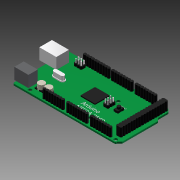
# Autodesk Inventor part: ArduinoMEGA2560
Saved by Autodesk Inventor 2012 (Build 160160000, 160)
## iProperties
Created: 2012-05-11
Part Number: ArduinoMEGA2560
Material: ABS Plastic
Document SubType Name: Modeling
Mass: 17.2903 g
Surface Area: 176.309 cm^2
Volume: 16.3116 cm^3
Density: 1.06 g/cm^3
Autodesk Inventor part; units mm, degrees
(part 1 of 2)
ref_plane "YZ Plane" through (0, 0, 0) normal (1, 0, 0) x (0, 1, 0)
ref_plane "XZ Plane" through (0, 0, 0) normal (0, 1, 0) x (-1, 0, 0)
sketch "Sketch1" plane through (0, 0, 0) normal (0, 0, 1) x (1, 0, 0)
  line L0 (96.5199, 53.3399) -> (99.0599, 50.7999)
  line L1 (99.0599, 40.6399) -> (101.5999, 38.0999)
  line L2 (101.5999, 38.0999) -> (101.5999, 3.81)
  line L3 (101.5999, 3.81) -> (99.0599, 1.27)
  line L4 (99.0599, 1.27) -> (99.0599, 1)
  arc A0 (98.0599, 0) -> (99.0599, 1) centre (98.0599, 1) ccw
  line L5 (98.0599, 0) -> (1, 0)
  arc A1 (0, 1) -> (1, 0) centre (1, 1) ccw
  line L6 (0, 1) -> (0, 52.3399)
  arc A2 (1, 53.3399) -> (0, 52.3399) centre (1, 52.3399) ccw
  line L7 (1, 53.3399) -> (96.5199, 53.3399)
  line L8 (99.0599, 50.7999) -> (99.0599, 40.6399)
  circle A3 centre (96.52, 2.54) radius 1.6
  circle A4 centre (15.24, 50.7999) radius 1.6
  circle A5 centre (90.17, 50.7999) radius 1.6
  circle A6 centre (13.97, 2.54) radius 1.6
  circle A7 centre (66.04, 35.5599) radius 1.6
  circle A8 centre (66.04, 7.62) radius 1.6
  point P0 (0, 0)
  dimension "d51" = 3.2
  dimension "d52" = 53.3399
  dimension "d53" = 101.5999
  dimension "d56" = 13.97
  dimension "d57" = 15.24
  dimension "d58" = 66.04
  dimension "d59" = 90.17
  dimension "d60" = 96.5199
  dimension "d61" = 2.54
  dimension "d62" = 50.7999
  dimension "d63" = 7.62
  dimension "d64" = 27.9399
  dimension "d65" = 98.0599
  dimension "d66" = 1
  dimension "d67" = 45
  dimension "d68" = 2.54
  dimension "d69" = 2.54
  dimension "d73" = 1.27
  dimension "d74" = 12.7
  constraints: 18 end point, 9 centre point, 7 equal radius, 7 tangent, 6 point on circle, 2 horizontal alignment, 2 parallel, 2 point on line, 1 horizontal, 1 perpendicular, 1 vertical, 1 vertical alignment
  measures "d51" diameter of A4
  measures "d52" distance between parallel lines of L5 L7
  measures "d53" distance between parallel lines of L2 L6
  measures "d56" distance from line of A6.centre L6
  measures "d57" distance from line of A4.centre L6
  measures "d58" distance from line of A7.centre L6
  measures "d59" distance from line of A5.centre L6
  measures "d60" distance from line of A3.centre L6
  measures "d61" distance from line of A6.centre L5
  measures "d62" distance from line of A4.centre L5
  measures "d63" distance from line of L5 A8.centre
  measures "d64" distance of A7.centre A8.centre
  measures "d65" distance from line of L6 A0.centre
  measures "d66" radius of A0
  measures "d67" angle of L7 L0
  measures "d68" horizontal distance of L0.start L0.end
  measures "d69" horizontal distance of L1.start L1.end
  measures "d73" distance from line of L3.end L5
  measures "d74" distance from line of L7 L1.start
extrude "PCB" add sketch "Sketch1" against normal blind 1.6
sketch "Sketch3" plane through (0, 0, 0) normal (0, 0, 1) x (1, 0, 0)
  arc A0 (21.844, 24.257) -> (21.844, 27.813) centre (21.844, 26.035) ccw
  arc A1 (21.844, 23.749) -> (21.844, 28.321) centre (21.844, 26.035) ccw
  arc A2 (14.986, 28.321) -> (14.986, 23.749) centre (14.986, 26.035) ccw
  arc A3 (14.986, 27.813) -> (14.986, 24.257) centre (14.986, 26.035) ccw
  line L0 (14.986, 24.257) -> (21.844, 24.257)
  line L1 (21.844, 27.813) -> (14.986, 27.813)
  line L2 (14.986, 23.749) -> (21.844, 23.749)
  line L3 (21.844, 28.321) -> (14.986, 28.321)
  line L4 (97.155, 6.35) -> (93.345, 6.35)
  arc A4 (97.155, 8.8519) -> (97.155, 8.9281) centre (97.155, 8.89) ccw
  line L5 (97.155, 8.89) -> (93.345, 8.89)
  line L6 (97.155, 11.43) -> (93.345, 11.43)
  line L7 (97.155, 13.97) -> (93.345, 13.97)
  line L8 (97.155, 16.51) -> (93.345, 16.51)
  line L9 (97.155, 19.05) -> (93.345, 19.05)
  line L10 (97.155, 21.59) -> (93.345, 21.59)
  line L11 (97.155, 24.13) -> (93.345, 24.13)
  line L12 (97.155, 26.67) -> (93.345, 26.67)
  line L13 (97.155, 29.21) -> (93.345, 29.21)
  line L14 (97.155, 31.75) -> (93.345, 31.75)
  line L15 (97.155, 34.29) -> (93.345, 34.29)
  line L16 (97.155, 36.83) -> (93.345, 36.83)
  line L17 (97.155, 39.37) -> (93.345, 39.37)
  line L18 (97.155, 41.91) -> (93.345, 41.91)
  line L19 (97.155, 44.45) -> (93.345, 44.45)
  line L20 (97.155, 46.99) -> (93.345, 46.99)
  line L21 (97.155, 49.53) -> (93.345, 49.53)
  line L22 (93.345, 36.83) -> (92.71, 36.195)
  line L23 (92.71, 34.925) -> (92.71, 36.195)
  line L24 (93.345, 34.29) -> (92.71, 34.925)
  line L25 (93.345, 34.29) -> (92.71, 33.655)
  line L26 (92.71, 32.385) -> (92.71, 33.655)
  line L27 (93.345, 31.75) -> (92.71, 32.385)
  line L28 (93.345, 31.75) -> (92.71, 31.115)
  line L29 (92.71, 29.845) -> (92.71, 31.115)
  line L30 (93.345, 29.21) -> (92.71, 29.845)
  line L31 (93.345, 29.21) -> (92.71, 28.575)
  line L32 (92.71, 27.305) -> (92.71, 28.575)
  line L33 (93.345, 26.67) -> (92.71, 27.305)
  line L34 (93.345, 26.67) -> (92.71, 26.035)
  line L35 (92.71, 24.765) -> (92.71, 26.035)
  line L36 (93.345, 24.13) -> (92.71, 24.765)
  line L37 (93.345, 24.13) -> (92.71, 23.495)
  line L38 (92.71, 22.225) -> (92.71, 23.495)
  line L39 (93.345, 21.59) -> (92.71, 22.225)
  line L40 (93.345, 21.59) -> (92.71, 20.955)
  line L41 (92.71, 19.685) -> (92.71, 20.955)
  line L42 (93.345, 19.05) -> (92.71, 19.685)
  line L43 (93.345, 19.05) -> (92.71, 18.415)
  line L44 (92.71, 17.145) -> (92.71, 18.415)
  line L45 (93.345, 16.51) -> (92.71, 17.145)
  line L46 (92.71, 15.875) -> (93.345, 16.51)
  line L47 (92.71, 15.875) -> (92.71, 14.605)
  line L48 (93.345, 13.97) -> (92.71, 14.605)
  line L49 (92.71, 13.335) -> (93.345, 13.97)
  line L50 (92.71, 13.335) -> (92.71, 12.065)
  line L51 (93.345, 11.43) -> (92.71, 12.065)
  line L52 (93.345, 11.43) -> (92.71, 10.795)
  line L53 (92.71, 9.525) -> (92.71, 10.795)
  line L54 (93.345, 8.89) -> (92.71, 9.525)
  line L55 (93.345, 8.89) -> (92.71, 8.255)
  line L56 (92.71, 6.985) -> (92.71, 8.255)
  line L57 (93.345, 6.35) -> (92.71, 6.985)
  line L58 (97.79, 6.985) -> (97.155, 6.35)
  line L59 (97.79, 6.985) -> (97.79, 8.255)
  arc A5 (97.1819, 8.9169) -> (97.1281, 8.8631) centre (97.155, 8.89) ccw
  line L60 (97.155, 8.89) -> (97.79, 8.255)
  arc A6 (97.1281, 8.8631) -> (97.1819, 8.8631) centre (97.155, 8.89) ccw
  line L61 (97.79, 9.525) -> (97.155, 8.89)
  line L62 (97.79, 9.525) -> (97.79, 10.795)
  line L63 (97.155, 11.43) -> (97.79, 10.795)
  line L64 (97.79, 12.065) -> (97.155, 11.43)
  line L65 (97.79, 12.065) -> (97.79, 13.335)
  line L66 (97.155, 13.97) -> (97.79, 13.335)
  line L67 (97.79, 14.605) -> (97.155, 13.97)
  line L68 (97.79, 14.605) -> (97.79, 15.875)
  line L69 (97.155, 16.51) -> (97.79, 15.875)
  line L70 (97.79, 17.145) -> (97.155, 16.51)
  line L71 (97.79, 17.145) -> (97.79, 18.415)
  line L72 (97.155, 19.05) -> (97.79, 18.415)
  line L73 (97.79, 19.685) -> (97.155, 19.05)
  line L74 (97.79, 19.685) -> (97.79, 20.955)
  line L75 (97.155, 21.59) -> (97.79, 20.955)
  line L76 (97.155, 21.59) -> (97.79, 22.225)
  line L77 (97.79, 23.495) -> (97.79, 22.225)
  line L78 (97.155, 24.13) -> (97.79, 23.495)
  line L79 (97.79, 24.765) -> (97.155, 24.13)
  line L80 (97.79, 26.035) -> (97.79, 24.765)
  line L81 (97.155, 26.67) -> (97.79, 26.035)
  line L82 (97.79, 27.305) -> (97.155, 26.67)
  line L83 (97.79, 28.575) -> (97.79, 27.305)
  line L84 (97.155, 29.21) -> (97.79, 28.575)
  line L85 (97.79, 29.845) -> (97.155, 29.21)
  line L86 (97.79, 31.115) -> (97.79, 29.845)
  line L87 (97.155, 31.75) -> (97.79, 31.115)
  line L88 (97.79, 32.385) -> (97.155, 31.75)
  line L89 (97.79, 33.655) -> (97.79, 32.385)
  line L90 (97.155, 34.29) -> (97.79, 33.655)
  line L91 (97.79, 34.925) -> (97.155, 34.29)
  line L92 (97.79, 36.195) -> (97.79, 34.925)
  line L93 (97.155, 36.83) -> (97.79, 36.195)
  line L94 (97.79, 37.465) -> (97.155, 36.83)
  line L95 (97.79, 38.735) -> (97.79, 37.465)
  line L96 (97.155, 39.37) -> (97.79, 38.735)
  line L97 (97.79, 40.005) -> (97.155, 39.37)
  line L98 (97.79, 41.275) -> (97.79, 40.005)
  line L99 (97.155, 41.91) -> (97.79, 41.275)
  line L100 (97.79, 42.545) -> (97.155, 41.91)
  line L101 (97.79, 43.815) -> (97.79, 42.545)
  line L102 (97.155, 44.45) -> (97.79, 43.815)
  line L103 (97.79, 45.085) -> (97.155, 44.45)
  line L104 (97.79, 46.355) -> (97.79, 45.085)
  line L105 (97.155, 46.99) -> (97.79, 46.355)
  line L106 (97.79, 47.625) -> (97.155, 46.99)
  line L107 (97.79, 48.895) -> (97.79, 47.625)
  line L108 (97.155, 49.53) -> (97.79, 48.895)
  line L109 (97.79, 50.165) -> (97.155, 49.53)
  line L110 (97.79, 51.435) -> (97.79, 50.165)
  line L111 (97.155, 52.07) -> (97.79, 51.435)
  line L112 (93.345, 52.07) -> (97.155, 52.07)
  line L113 (92.71, 37.465) -> (93.345, 36.83)
  line L114 (92.71, 38.735) -> (92.71, 37.465)
  line L115 (93.345, 39.37) -> (92.71, 38.735)
  line L116 (92.71, 40.005) -> (93.345, 39.37)
  line L117 (92.71, 41.275) -> (92.71, 40.005)
  line L118 (93.345, 41.91) -> (92.71, 41.275)
  line L119 (92.71, 42.545) -> (93.345, 41.91)
  line L120 (92.71, 43.815) -> (92.71, 42.545)
  line L121 (93.345, 44.45) -> (92.71, 43.815)
  line L122 (92.71, 45.085) -> (93.345, 44.45)
  line L123 (92.71, 46.355) -> (92.71, 45.085)
  line L124 (93.345, 46.99) -> (92.71, 46.355)
  line L125 (92.71, 47.625) -> (93.345, 46.99)
  line L126 (92.71, 48.895) -> (92.71, 47.625)
  line L127 (93.345, 49.53) -> (92.71, 48.895)
  line L128 (92.71, 50.165) -> (93.345, 49.53)
  line L129 (92.71, 51.435) -> (92.71, 50.165)
  line L130 (93.345, 52.07) -> (92.71, 51.435)
  line L131 (8.763, 27.3304) -> (9.525, 27.3304)
  line L132 (8.763, 24.4348) -> (8.763, 27.3304)
  line L133 (9.525, 24.4348) -> (8.763, 24.4348)
  line L134 (9.525, 27.3304) -> (9.525, 24.4348)
  line L135 (26.543, 16.764) -> (29.337, 16.764)
  line L136 (26.289, 14.986) -> (26.289, 16.51)
  line L137 (29.591, 14.986) -> (29.591, 16.51)
  arc A7 (29.337, 14.732) -> (29.591, 14.986) centre (29.337, 14.986) ccw
  arc A8 (26.289, 14.986) -> (26.543, 14.732) centre (26.543, 14.986) ccw
  arc A9 (26.543, 16.764) -> (26.289, 16.51) centre (26.543, 16.51) ccw
  arc A10 (29.591, 16.51) -> (29.337, 16.764) centre (29.337, 16.51) ccw
  line L138 (29.337, 14.732) -> (26.543, 14.732)
  arc A11 (74.168, 26.74) -> (74.168, 29.14) centre (74.168, 27.94) ccw
  arc A12 (74.168, 29.14) -> (74.168, 26.74) centre (74.168, 27.94) ccw
  arc A13 (74.168, 26.44) -> (74.168, 29.44) centre (74.168, 27.94) ccw
  arc A14 (74.168, 29.44) -> (74.168, 26.44) centre (74.168, 27.94) ccw
  line L139 (76.168, 26.94) -> (76.168, 25.09)
  line L140 (76.168, 28.94) -> (76.168, 30.79)
  line L141 (72.168, 28.94) -> (72.168, 30.79)
  line L142 (72.168, 25.09) -> (72.168, 26.94)
  line L143 (76.168, 26.94) -> (76.368, 26.94)
  line L144 (75.968, 26.94) -> (76.168, 26.94)
  line L145 (75.968, 28.94) -> (75.968, 26.94)
  line L146 (76.168, 28.94) -> (75.968, 28.94)
  line L147 (76.368, 28.94) -> (76.168, 28.94)
  line L148 (76.368, 26.94) -> (76.368, 28.94)
  line L149 (72.168, 26.94) -> (72.368, 26.94)
  line L150 (71.968, 26.94) -> (72.168, 26.94)
  line L151 (71.968, 28.94) -> (71.968, 26.94)
  line L152 (72.168, 28.94) -> (71.968, 28.94)
  line L153 (72.368, 28.94) -> (72.168, 28.94)
  line L154 (72.368, 26.94) -> (72.368, 28.94)
  line L155 (74.668, 24.84) -> (74.668, 25.09)
  line L156 (73.668, 24.84) -> (74.668, 24.84)
  line L157 (73.668, 25.09) -> (73.668, 24.84)
  line L158 (74.668, 25.09) -> (76.168, 25.09)
  line L159 (72.168, 25.09) -> (73.668, 25.09)
  line L160 (76.168, 30.79) -> (72.168, 30.79)
  line L161 (45.085, 52.07) -> (46.355, 52.07)
  line L162 (46.99, 51.435) -> (46.355, 52.07)
  line L163 (46.355, 49.53) -> (46.99, 50.165)
  line L164 (44.45, 51.435) -> (45.085, 52.07)
  line L165 (44.45, 50.165) -> (44.45, 51.435)
  line L166 (45.085, 49.53) -> (44.45, 50.165)
  line L167 (46.355, 49.53) -> (45.085, 49.53)
  line L168 (62.865, 52.07) -> (64.135, 52.07)
  line L169 (64.77, 51.435) -> (64.135, 52.07)
  line L170 (64.135, 49.53) -> (64.77, 50.165)
  line L171 (64.77, 50.165) -> (64.77, 51.435)
  line L172 (61.595, 52.07) -> (62.23, 51.435)
  line L173 (60.325, 52.07) -> (61.595, 52.07)
  line L174 (59.69, 51.435) -> (60.325, 52.07)
  line L175 (59.69, 50.165) -> (59.69, 51.435)
  line L176 (60.325, 49.53) -> (59.69, 50.165)
  line L177 (61.595, 49.53) -> (60.325, 49.53)
  line L178 (62.23, 50.165) -> (61.595, 49.53)
  line L179 (62.23, 51.435) -> (62.865, 52.07)
  line L180 (62.23, 50.165) -> (62.23, 51.435)
  line L181 (62.865, 49.53) -> (62.23, 50.165)
  line L182 (64.135, 49.53) -> (62.865, 49.53)
  line L183 (55.245, 52.07) -> (56.515, 52.07)
  line L184 (57.15, 51.435) -> (56.515, 52.07)
  line L185 (59.055, 52.07) -> (59.69, 51.435)
  line L186 (57.785, 52.07) -> (59.055, 52.07)
  line L187 (57.15, 51.435) -> (57.785, 52.07)
  line L188 (57.15, 50.165) -> (57.15, 51.435)
  line L189 (57.785, 49.53) -> (57.15, 50.165)
  line L190 (59.055, 49.53) -> (57.785, 49.53)
  line L191 (59.69, 50.165) -> (59.055, 49.53)
  line L192 (53.975, 52.07) -> (54.61, 51.435)
  line L193 (52.705, 52.07) -> (53.975, 52.07)
  line L194 (52.07, 51.435) -> (52.705, 52.07)
  line L195 (52.07, 50.165) -> (52.07, 51.435)
  line L196 (52.705, 49.53) -> (52.07, 50.165)
  line L197 (53.975, 49.53) -> (52.705, 49.53)
  line L198 (54.61, 50.165) -> (53.975, 49.53)
  line L199 (54.61, 51.435) -> (55.245, 52.07)
  line L200 (54.61, 50.165) -> (54.61, 51.435)
  line L201 (55.245, 49.53) -> (54.61, 50.165)
  line L202 (56.515, 49.53) -> (55.245, 49.53)
  line L203 (47.625, 52.07) -> (48.895, 52.07)
  line L204 (49.53, 51.435) -> (48.895, 52.07)
  line L205 (48.895, 49.53) -> (49.53, 50.165)
  line L206 (51.435, 52.07) -> (52.07, 51.435)
  line L207 (50.165, 52.07) -> (51.435, 52.07)
  line L208 (49.53, 51.435) -> (50.165, 52.07)
  line L209 (49.53, 50.165) -> (49.53, 51.435)
  line L210 (50.165, 49.53) -> (49.53, 50.165)
  line L211 (51.435, 49.53) -> (50.165, 49.53)
  line L212 (52.07, 50.165) -> (51.435, 49.53)
  line L213 (46.99, 51.435) -> (47.625, 52.07)
  line L214 (46.99, 50.165) -> (46.99, 51.435)
  line L215 (47.625, 49.53) -> (46.99, 50.165)
  line L216 (48.895, 49.53) -> (47.625, 49.53)
  line L217 (46.355, 1.27) -> (45.085, 1.27)
  line L218 (44.45, 1.905) -> (45.085, 1.27)
  line L219 (45.085, 3.81) -> (44.45, 3.175)
  line L220 (46.99, 1.905) -> (46.355, 1.27)
  line L221 (46.99, 3.175) -> (46.99, 1.905)
  line L222 (46.355, 3.81) -> (46.99, 3.175)
  line L223 (45.085, 3.81) -> (46.355, 3.81)
  line L224 (28.575, 1.27) -> (27.305, 1.27)
  line L225 (26.67, 1.905) -> (27.305, 1.27)
  line L226 (27.305, 3.81) -> (26.67, 3.175)
  line L227 (26.67, 3.175) -> (26.67, 1.905)
  line L228 (29.845, 1.27) -> (29.21, 1.905)
  line L229 (31.115, 1.27) -> (29.845, 1.27)
  line L230 (31.75, 1.905) -> (31.115, 1.27)
  line L231 (31.75, 3.175) -> (31.75, 1.905)
  line L232 (31.115, 3.81) -> (31.75, 3.175)
  line L233 (29.845, 3.81) -> (31.115, 3.81)
  line L234 (29.21, 3.175) -> (29.845, 3.81)
  line L235 (29.21, 1.905) -> (28.575, 1.27)
  line L236 (29.21, 3.175) -> (29.21, 1.905)
  line L237 (28.575, 3.81) -> (29.21, 3.175)
  line L238 (27.305, 3.81) -> (28.575, 3.81)
  line L239 (36.195, 1.27) -> (34.925, 1.27)
  line L240 (34.29, 1.905) -> (34.925, 1.27)
  line L241 (34.925, 3.81) -> (34.29, 3.175)
  line L242 (32.385, 1.27) -> (31.75, 1.905)
  line L243 (33.655, 1.27) -> (32.385, 1.27)
  line L244 (34.29, 1.905) -> (33.655, 1.27)
  line L245 (34.29, 3.175) -> (34.29, 1.905)
  line L246 (33.655, 3.81) -> (34.29, 3.175)
  line L247 (32.385, 3.81) -> (33.655, 3.81)
  line L248 (31.75, 3.175) -> (32.385, 3.81)
  line L249 (37.465, 1.27) -> (36.83, 1.905)
  line L250 (38.735, 1.27) -> (37.465, 1.27)
  line L251 (39.37, 1.905) -> (38.735, 1.27)
  line L252 (39.37, 3.175) -> (39.37, 1.905)
  line L253 (38.735, 3.81) -> (39.37, 3.175)
  line L254 (37.465, 3.81) -> (38.735, 3.81)
  line L255 (36.83, 3.175) -> (37.465, 3.81)
  line L256 (36.83, 1.905) -> (36.195, 1.27)
  line L257 (36.83, 3.175) -> (36.83, 1.905)
  line L258 (36.195, 3.81) -> (36.83, 3.175)
  line L259 (34.925, 3.81) -> (36.195, 3.81)
  line L260 (43.815, 1.27) -> (42.545, 1.27)
  line L261 (41.91, 1.905) -> (42.545, 1.27)
  line L262 (42.545, 3.81) -> (41.91, 3.175)
  line L263 (40.005, 1.27) -> (39.37, 1.905)
  line L264 (41.275, 1.27) -> (40.005, 1.27)
  line L265 (41.91, 1.905) -> (41.275, 1.27)
  line L266 (41.91, 3.175) -> (41.91, 1.905)
  line L267 (41.275, 3.81) -> (41.91, 3.175)
  line L268 (40.005, 3.81) -> (41.275, 3.81)
  line L269 (39.37, 3.175) -> (40.005, 3.81)
  line L270 (44.45, 1.905) -> (43.815, 1.27)
  line L271 (44.45, 3.175) -> (44.45, 1.905)
  line L272 (43.815, 3.81) -> (44.45, 3.175)
  line L273 (42.545, 3.81) -> (43.815, 3.81)
  arc A15 (26.477, 6.194) -> (26.477, 12.094) centre (25.5268, 9.144) ccw
  arc A16 (24.577, 12.094) -> (24.577, 6.194) centre (25.5272, 9.144) ccw
  line L274 (28.777, 5.894) -> (26.477, 5.894)
  line L275 (28.777, 10.694) -> (28.777, 5.894)
  line L276 (27.077, 12.394) -> (28.777, 10.694)
  line L277 (26.477, 12.394) -> (27.077, 12.394)
  line L278 (23.977, 12.394) -> (24.577, 12.394)
  line L279 (22.277, 10.694) -> (23.977, 12.394)
  line L280 (22.277, 5.894) -> (22.277, 10.694)
  line L281 (24.577, 5.894) -> (22.277, 5.894)
  arc A17 (19.365, 6.194) -> (19.365, 12.094) centre (18.4148, 9.144) ccw
  arc A18 (17.465, 12.094) -> (17.465, 6.194) centre (18.4152, 9.144) ccw
  line L282 (21.665, 5.894) -> (19.365, 5.894)
  line L283 (21.665, 10.694) -> (21.665, 5.894)
  line L284 (19.965, 12.394) -> (21.665, 10.694)
  line L285 (19.365, 12.394) -> (19.965, 12.394)
  line L286 (16.865, 12.394) -> (17.465, 12.394)
  line L287 (15.165, 10.694) -> (16.865, 12.394)
  arc A19 (15.1396, 5.894) -> (15.1904, 5.894) centre (15.165, 5.894) ccw
  line L288 (15.165, 5.894) -> (15.165, 10.694)
  arc A20 (15.165, 5.9194) -> (15.1396, 5.894) centre (15.165, 5.894) ccw
  line L289 (17.465, 5.894) -> (15.165, 5.894)
  line L290 (42.291, 49.53) -> (41.021, 49.53)
  line L291 (40.386, 50.165) -> (41.021, 49.53)
  line L292 (41.021, 52.07) -> (40.386, 51.435)
  line L293 (42.926, 50.165) -> (42.291, 49.53)
  line L294 (42.926, 51.435) -> (42.926, 50.165)
  line L295 (42.291, 52.07) -> (42.926, 51.435)
  line L296 (41.021, 52.07) -> (42.291, 52.07)
  line L297 (19.431, 49.53) -> (18.161, 49.53)
  line L298 (17.526, 50.165) -> (18.161, 49.53)
  line L299 (18.161, 52.07) -> (17.526, 51.435)
  line L300 (17.526, 51.435) -> (17.526, 50.165)
  line L301 (20.701, 49.53) -> (20.066, 50.165)
  line L302 (21.971, 49.53) -> (20.701, 49.53)
  line L303 (22.606, 50.165) -> (21.971, 49.53)
  line L304 (22.606, 51.435) -> (22.606, 50.165)
  line L305 (21.971, 52.07) -> (22.606, 51.435)
  line L306 (20.701, 52.07) -> (21.971, 52.07)
  line L307 (20.066, 51.435) -> (20.701, 52.07)
  line L308 (20.066, 50.165) -> (19.431, 49.53)
  line L309 (20.066, 51.435) -> (20.066, 50.165)
  line L310 (19.431, 52.07) -> (20.066, 51.435)
  line L311 (18.161, 52.07) -> (19.431, 52.07)
  line L312 (27.051, 49.53) -> (25.781, 49.53)
  line L313 (25.146, 50.165) -> (25.781, 49.53)
  line L314 (25.781, 52.07) -> (25.146, 51.435)
  line L315 (23.241, 49.53) -> (22.606, 50.165)
  line L316 (24.511, 49.53) -> (23.241, 49.53)
  line L317 (25.146, 50.165) -> (24.511, 49.53)
  line L318 (25.146, 51.435) -> (25.146, 50.165)
  line L319 (24.511, 52.07) -> (25.146, 51.435)
  line L320 (23.241, 52.07) -> (24.511, 52.07)
  line L321 (22.606, 51.435) -> (23.241, 52.07)
  line L322 (28.321, 49.53) -> (27.686, 50.165)
  line L323 (29.591, 49.53) -> (28.321, 49.53)
  line L324 (30.226, 50.165) -> (29.591, 49.53)
  line L325 (30.226, 51.435) -> (30.226, 50.165)
  line L326 (29.591, 52.07) -> (30.226, 51.435)
  line L327 (28.321, 52.07) -> (29.591, 52.07)
  line L328 (27.686, 51.435) -> (28.321, 52.07)
  line L329 (27.686, 50.165) -> (27.051, 49.53)
  line L330 (27.686, 51.435) -> (27.686, 50.165)
  line L331 (27.051, 52.07) -> (27.686, 51.435)
  line L332 (25.781, 52.07) -> (27.051, 52.07)
  line L333 (34.671, 49.53) -> (33.401, 49.53)
  line L334 (32.766, 50.165) -> (33.401, 49.53)
  line L335 (33.401, 52.07) -> (32.766, 51.435)
  line L336 (30.861, 49.53) -> (30.226, 50.165)
  line L337 (32.131, 49.53) -> (30.861, 49.53)
  line L338 (32.766, 50.165) -> (32.131, 49.53)
  line L339 (32.766, 51.435) -> (32.766, 50.165)
  line L340 (32.131, 52.07) -> (32.766, 51.435)
  line L341 (30.861, 52.07) -> (32.131, 52.07)
  line L342 (30.226, 51.435) -> (30.861, 52.07)
  line L343 (35.941, 49.53) -> (35.306, 50.165)
  line L344 (37.211, 49.53) -> (35.941, 49.53)
  line L345 (37.846, 50.165) -> (37.211, 49.53)
  line L346 (37.846, 51.435) -> (37.846, 50.165)
  line L347 (37.211, 52.07) -> (37.846, 51.435)
  line L348 (35.941, 52.07) -> (37.211, 52.07)
  line L349 (35.306, 51.435) -> (35.941, 52.07)
  line L350 (35.306, 50.165) -> (34.671, 49.53)
  line L351 (35.306, 51.435) -> (35.306, 50.165)
  line L352 (34.671, 52.07) -> (35.306, 51.435)
  line L353 (33.401, 52.07) -> (34.671, 52.07)
  line L354 (38.481, 49.53) -> (37.846, 50.165)
  line L355 (39.751, 49.53) -> (38.481, 49.53)
  line L356 (40.386, 50.165) -> (39.751, 49.53)
  line L357 (40.386, 51.435) -> (40.386, 50.165)
  line L358 (39.751, 52.07) -> (40.386, 51.435)
  line L359 (38.481, 52.07) -> (39.751, 52.07)
  line L360 (37.846, 51.435) -> (38.481, 52.07)
  line L361 (22.098, 39.243) -> (22.098, 40.513)
  line L362 (22.098, 41.783) -> (22.098, 43.053)
  line L363 (17.653, 43.688) -> (21.463, 43.688)
  line L364 (17.653, 41.148) -> (21.463, 41.148)
  line L365 (17.018, 43.053) -> (17.653, 43.688)
  line L366 (17.018, 41.783) -> (17.018, 43.053)
  line L367 (17.653, 41.148) -> (17.018, 41.783)
  line L368 (17.018, 40.513) -> (17.653, 41.148)
  line L369 (17.018, 39.243) -> (17.018, 40.513)
  line L370 (17.653, 38.608) -> (17.018, 39.243)
  line L371 (21.463, 38.608) -> (17.653, 38.608)
  line L372 (22.098, 43.053) -> (21.463, 43.688)
  line L373 (21.463, 41.148) -> (22.098, 41.783)
  line L374 (22.098, 40.513) -> (21.463, 41.148)
  line L375 (21.463, 38.608) -> (22.098, 39.243)
  line L376 (16.383, 48.768) -> (15.113, 48.768)
  line L377 (14.478, 44.323) -> (14.478, 48.133)
  line L378 (15.113, 43.688) -> (14.478, 44.323)
  line L379 (16.383, 43.688) -> (15.113, 43.688)
  line L380 (17.018, 44.323) -> (16.383, 43.688)
  line L381 (15.113, 48.768) -> (14.478, 48.133)
  line L382 (17.018, 48.133) -> (16.383, 48.768)
  line L383 (21.463, 48.768) -> (20.193, 48.768)
  line L384 (18.923, 48.768) -> (17.653, 48.768)
  line L385 (17.018, 44.323) -> (17.018, 48.133)
  line L386 (19.558, 44.323) -> (19.558, 48.133)
  line L387 (17.653, 43.688) -> (17.018, 44.323)
  line L388 (18.923, 43.688) -> (17.653, 43.688)
  line L389 (19.558, 44.323) -> (18.923, 43.688)
  line L390 (20.193, 43.688) -> (19.558, 44.323)
  line L391 (21.463, 43.688) -> (20.193, 43.688)
  line L392 (22.098, 44.323) -> (21.463, 43.688)
  line L393 (22.098, 48.133) -> (22.098, 44.323)
  line L394 (17.653, 48.768) -> (17.018, 48.133)
  line L395 (19.558, 48.133) -> (18.923, 48.768)
  line L396 (20.193, 48.768) -> (19.558, 48.133)
  line L397 (22.098, 48.133) -> (21.463, 48.768)
  line L398 (62.357, 26.035) -> (62.357, 24.765)
  line L399 (66.802, 24.13) -> (62.992, 24.13)
  line L400 (67.437, 24.765) -> (66.802, 24.13)
  line L401 (67.437, 26.035) -> (67.437, 24.765)
  line L402 (66.802, 26.67) -> (67.437, 26.035)
  line L403 (62.357, 24.765) -> (62.992, 24.13)
  line L404 (62.992, 26.67) -> (62.357, 26.035)
  line L405 (62.357, 31.115) -> (62.357, 29.845)
  line L406 (62.357, 28.575) -> (62.357, 27.305)
  line L407 (66.802, 26.67) -> (62.992, 26.67)
  line L408 (66.802, 29.21) -> (62.992, 29.21)
  line L409 (67.437, 27.305) -> (66.802, 26.67)
  line L410 (67.437, 28.575) -> (67.437, 27.305)
  line L411 (66.802, 29.21) -> (67.437, 28.575)
  line L412 (67.437, 29.845) -> (66.802, 29.21)
  line L413 (67.437, 31.115) -> (67.437, 29.845)
  line L414 (66.802, 31.75) -> (67.437, 31.115)
  line L415 (62.992, 31.75) -> (66.802, 31.75)
  line L416 (62.357, 27.305) -> (62.992, 26.67)
  line L417 (62.992, 29.21) -> (62.357, 28.575)
  line L418 (62.357, 29.845) -> (62.992, 29.21)
  line L419 (62.992, 31.75) -> (62.357, 31.115)
  arc A21 (19.2056, 19.8904) -> (19.2056, 20.8904) centre (19.2056, 20.3904) ccw
  arc A22 (19.2056, 20.8904) -> (19.2056, 19.8904) centre (19.2056, 20.3904) ccw
  arc A23 (20.041, 22.635) -> (19.716, 22.96) centre (19.716, 22.635) ccw
  arc A24 (19.716, 19.71) -> (20.041, 20.035) centre (19.716, 20.035) ccw
  arc A25 (16.791, 20.035) -> (17.116, 19.71) centre (17.116, 20.035) ccw
  arc A26 (17.116, 22.96) -> (16.791, 22.635) centre (17.116, 22.635) ccw
  line L420 (19.716, 19.71) -> (17.116, 19.71)
  line L421 (17.116, 22.96) -> (19.716, 22.96)
  arc A27 (18.339, 32.8818) -> (18.339, 33.5142) centre (18.339, 33.198) ccw
  arc A28 (18.339, 33.5142) -> (18.339, 32.8818) centre (18.339, 33.198) ccw
  line L422 (17.7565, 32.298) -> (22.439, 32.298)
  line L423 (17.439, 32.6155) -> (17.7565, 32.298)
  line L424 (17.439, 37.298) -> (17.439, 32.6155)
  line L425 (22.439, 37.298) -> (17.439, 37.298)
  line L426 (22.439, 32.298) -> (22.439, 37.298)
  arc A29 (44.8, 34.0965) -> (44.8, 34.5963) centre (44.8, 34.3464) ccw
  arc A30 (44.8, 34.5963) -> (44.8, 34.0965) centre (44.8, 34.3464) ccw
  line L427 (43.8, 21.5964) -> (43.8, 34.5964)
  line L428 (44.05, 21.3464) -> (43.8, 21.5964)
  line L429 (57.55, 21.3464) -> (44.05, 21.3464)
  line L430 (57.8, 21.5964) -> (57.55, 21.3464)
  line L431 (57.8, 35.0964) -> (57.8, 21.5964)
  line L432 (57.55, 35.3464) -> (57.8, 35.0964)
  line L433 (44.55, 35.3464) -> (57.55, 35.3464)
  line L434 (43.8, 34.5964) -> (44.55, 35.3464)
  line L435 (6.858, 14.5034) -> (6.858, 21.0566)
  line L436 (10.414, 14.5034) -> (6.858, 14.5034)
  line L437 (10.414, 21.0566) -> (10.414, 14.5034)
  line L438 (6.858, 21.0566) -> (10.414, 21.0566)
  line L439 (13.581, 46.728) -> (12.581, 46.728)
  line L440 (13.081, 45.728) -> (13.581, 46.728)
  line L441 (12.581, 46.728) -> (13.081, 45.728)
  line L442 (21.397, 3.794) -> (21.397, 1.794)
  line L443 (22.42, 2.794) -> (21.397, 3.794)
  line L444 (21.397, 1.794) -> (22.42, 2.794)
  line L445 (23.8506, 4.699) -> (19.3294, 4.699)
  line L446 (23.8506, 0.889) -> (19.3294, 0.889)
  line L447 (67.945, 52.07) -> (69.215, 52.07)
  line L448 (69.85, 51.435) -> (69.215, 52.07)
  line L449 (69.215, 49.53) -> (69.85, 50.165)
  line L450 (67.31, 51.435) -> (67.945, 52.07)
  line L451 (67.31, 50.165) -> (67.31, 51.435)
  line L452 (67.945, 49.53) -> (67.31, 50.165)
  line L453 (69.215, 49.53) -> (67.945, 49.53)
  line L454 (85.725, 52.07) -> (86.995, 52.07)
  line L455 (87.63, 51.435) -> (86.995, 52.07)
  line L456 (86.995, 49.53) -> (87.63, 50.165)
  line L457 (87.63, 50.165) -> (87.63, 51.435)
  line L458 (84.455, 52.07) -> (85.09, 51.435)
  line L459 (83.185, 52.07) -> (84.455, 52.07)
  line L460 (82.55, 51.435) -> (83.185, 52.07)
  line L461 (82.55, 50.165) -> (82.55, 51.435)
  line L462 (83.185, 49.53) -> (82.55, 50.165)
  line L463 (84.455, 49.53) -> (83.185, 49.53)
  line L464 (85.09, 50.165) -> (84.455, 49.53)
  line L465 (85.09, 51.435) -> (85.725, 52.07)
  line L466 (85.09, 50.165) -> (85.09, 51.435)
  line L467 (85.725, 49.53) -> (85.09, 50.165)
  line L468 (86.995, 49.53) -> (85.725, 49.53)
  line L469 (78.105, 52.07) -> (79.375, 52.07)
  line L470 (80.01, 51.435) -> (79.375, 52.07)
  line L471 (79.375, 49.53) -> (80.01, 50.165)
  line L472 (81.915, 52.07) -> (82.55, 51.435)
  line L473 (80.645, 52.07) -> (81.915, 52.07)
  line L474 (80.01, 51.435) -> (80.645, 52.07)
  line L475 (80.01, 50.165) -> (80.01, 51.435)
  line L476 (80.645, 49.53) -> (80.01, 50.165)
  line L477 (81.915, 49.53) -> (80.645, 49.53)
  line L478 (82.55, 50.165) -> (81.915, 49.53)
  line L479 (75.565, 52.07) -> (76.835, 52.07)
  line L480 (74.93, 51.435) -> (75.565, 52.07)
  line L481 (74.93, 50.165) -> (74.93, 51.435)
  line L482 (75.565, 49.53) -> (74.93, 50.165)
  line L483 (76.835, 49.53) -> (75.565, 49.53)
  line L484 (77.47, 50.165) -> (76.835, 49.53)
  line L485 (77.47, 51.435) -> (78.105, 52.07)
  line L486 (77.47, 50.165) -> (77.47, 51.435)
  line L487 (78.105, 49.53) -> (77.47, 50.165)
  line L488 (79.375, 49.53) -> (78.105, 49.53)
  line L489 (70.485, 52.07) -> (71.755, 52.07)
  line L490 (72.39, 51.435) -> (71.755, 52.07)
  line L491 (71.755, 49.53) -> (72.39, 50.165)
  line L492 (74.295, 52.07) -> (74.93, 51.435)
  line L493 (73.025, 52.07) -> (74.295, 52.07)
  line L494 (72.39, 51.435) -> (73.025, 52.07)
  line L495 (72.39, 50.165) -> (72.39, 51.435)
  line L496 (73.025, 49.53) -> (72.39, 50.165)
  line L497 (74.295, 49.53) -> (73.025, 49.53)
  line L498 (74.93, 50.165) -> (74.295, 49.53)
  line L499 (69.85, 51.435) -> (70.485, 52.07)
  line L500 (69.85, 50.165) -> (69.85, 51.435)
  line L501 (70.485, 49.53) -> (69.85, 50.165)
  line L502 (71.755, 49.53) -> (70.485, 49.53)
  line L503 (69.215, 1.27) -> (67.945, 1.27)
  line L504 (67.31, 1.905) -> (67.945, 1.27)
  line L505 (67.945, 3.81) -> (67.31, 3.175)
  line L506 (69.85, 1.905) -> (69.215, 1.27)
  line L507 (69.85, 3.175) -> (69.85, 1.905)
  line L508 (69.215, 3.81) -> (69.85, 3.175)
  line L509 (67.945, 3.81) -> (69.215, 3.81)
  line L510 (51.435, 1.27) -> (50.165, 1.27)
  line L511 (49.53, 1.905) -> (50.165, 1.27)
  line L512 (50.165, 3.81) -> (49.53, 3.175)
  line L513 (49.53, 3.175) -> (49.53, 1.905)
  line L514 (52.705, 1.27) -> (52.07, 1.905)
  line L515 (53.975, 1.27) -> (52.705, 1.27)
  line L516 (54.61, 1.905) -> (53.975, 1.27)
  line L517 (54.61, 3.175) -> (54.61, 1.905)
  line L518 (53.975, 3.81) -> (54.61, 3.175)
  line L519 (52.705, 3.81) -> (53.975, 3.81)
  line L520 (52.07, 3.175) -> (52.705, 3.81)
  line L521 (52.07, 1.905) -> (51.435, 1.27)
  line L522 (52.07, 3.175) -> (52.07, 1.905)
  line L523 (51.435, 3.81) -> (52.07, 3.175)
  line L524 (50.165, 3.81) -> (51.435, 3.81)
  line L525 (59.055, 1.27) -> (57.785, 1.27)
  line L526 (57.15, 1.905) -> (57.785, 1.27)
  line L527 (57.785, 3.81) -> (57.15, 3.175)
  line L528 (55.245, 1.27) -> (54.61, 1.905)
  line L529 (56.515, 1.27) -> (55.245, 1.27)
  line L530 (57.15, 1.905) -> (56.515, 1.27)
  line L531 (57.15, 3.175) -> (57.15, 1.905)
  line L532 (56.515, 3.81) -> (57.15, 3.175)
  line L533 (55.245, 3.81) -> (56.515, 3.81)
  line L534 (54.61, 3.175) -> (55.245, 3.81)
  line L535 (60.325, 1.27) -> (59.69, 1.905)
  line L536 (61.595, 1.27) -> (60.325, 1.27)
  line L537 (62.23, 1.905) -> (61.595, 1.27)
  line L538 (62.23, 3.175) -> (62.23, 1.905)
  line L539 (61.595, 3.81) -> (62.23, 3.175)
  line L540 (60.325, 3.81) -> (61.595, 3.81)
  line L541 (59.69, 3.175) -> (60.325, 3.81)
  line L542 (59.69, 1.905) -> (59.055, 1.27)
  line L543 (59.69, 3.175) -> (59.69, 1.905)
  line L544 (59.055, 3.81) -> (59.69, 3.175)
  line L545 (57.785, 3.81) -> (59.055, 3.81)
  line L546 (66.675, 1.27) -> (65.405, 1.27)
  line L547 (64.77, 1.905) -> (65.405, 1.27)
  line L548 (65.405, 3.81) -> (64.77, 3.175)
  line L549 (62.865, 1.27) -> (62.23, 1.905)
  line L550 (64.135, 1.27) -> (62.865, 1.27)
  line L551 (64.77, 1.905) -> (64.135, 1.27)
  line L552 (64.77, 3.175) -> (64.77, 1.905)
  line L553 (64.135, 3.81) -> (64.77, 3.175)
  line L554 (62.865, 3.81) -> (64.135, 3.81)
  line L555 (62.23, 3.175) -> (62.865, 3.81)
  line L556 (67.31, 1.905) -> (66.675, 1.27)
  line L557 (67.31, 3.175) -> (67.31, 1.905)
  line L558 (66.675, 3.81) -> (67.31, 3.175)
  line L559 (65.405, 3.81) -> (66.675, 3.81)
  line L560 (92.075, 1.27) -> (90.805, 1.27)
  line L561 (90.17, 1.905) -> (90.805, 1.27)
  line L562 (90.805, 3.81) -> (90.17, 3.175)
  line L563 (92.71, 1.905) -> (92.075, 1.27)
  line L564 (92.71, 3.175) -> (92.71, 1.905)
  line L565 (92.075, 3.81) -> (92.71, 3.175)
  line L566 (90.805, 3.81) -> (92.075, 3.81)
  line L567 (74.295, 1.27) -> (73.025, 1.27)
  line L568 (72.39, 1.905) -> (73.025, 1.27)
  line L569 (73.025, 3.81) -> (72.39, 3.175)
  line L570 (72.39, 3.175) -> (72.39, 1.905)
  line L571 (75.565, 1.27) -> (74.93, 1.905)
  line L572 (76.835, 1.27) -> (75.565, 1.27)
  line L573 (77.47, 1.905) -> (76.835, 1.27)
  line L574 (77.47, 3.175) -> (77.47, 1.905)
  line L575 (76.835, 3.81) -> (77.47, 3.175)
  line L576 (75.565, 3.81) -> (76.835, 3.81)
  line L577 (74.93, 3.175) -> (75.565, 3.81)
  line L578 (74.93, 1.905) -> (74.295, 1.27)
  line L579 (74.93, 3.175) -> (74.93, 1.905)
  line L580 (74.295, 3.81) -> (74.93, 3.175)
  line L581 (73.025, 3.81) -> (74.295, 3.81)
  line L582 (81.915, 1.27) -> (80.645, 1.27)
  line L583 (80.01, 1.905) -> (80.645, 1.27)
  line L584 (80.645, 3.81) -> (80.01, 3.175)
  line L585 (78.105, 1.27) -> (77.47, 1.905)
  line L586 (79.375, 1.27) -> (78.105, 1.27)
  line L587 (80.01, 1.905) -> (79.375, 1.27)
  line L588 (80.01, 3.175) -> (80.01, 1.905)
  line L589 (79.375, 3.81) -> (80.01, 3.175)
  line L590 (78.105, 3.81) -> (79.375, 3.81)
  line L591 (77.47, 3.175) -> (78.105, 3.81)
  line L592 (83.185, 1.27) -> (82.55, 1.905)
  line L593 (84.455, 1.27) -> (83.185, 1.27)
  line L594 (85.09, 1.905) -> (84.455, 1.27)
  line L595 (85.09, 3.175) -> (85.09, 1.905)
  line L596 (84.455, 3.81) -> (85.09, 3.175)
  line L597 (83.185, 3.81) -> (84.455, 3.81)
  line L598 (82.55, 3.175) -> (83.185, 3.81)
  line L599 (82.55, 1.905) -> (81.915, 1.27)
  line L600 (82.55, 3.175) -> (82.55, 1.905)
  line L601 (81.915, 3.81) -> (82.55, 3.175)
  line L602 (80.645, 3.81) -> (81.915, 3.81)
  line L603 (89.535, 1.27) -> (88.265, 1.27)
  line L604 (87.63, 1.905) -> (88.265, 1.27)
  line L605 (88.265, 3.81) -> (87.63, 3.175)
  line L606 (85.725, 1.27) -> (85.09, 1.905)
  line L607 (86.995, 1.27) -> (85.725, 1.27)
  line L608 (87.63, 1.905) -> (86.995, 1.27)
  line L609 (87.63, 3.175) -> (87.63, 1.905)
  line L610 (86.995, 3.81) -> (87.63, 3.175)
  line L611 (85.725, 3.81) -> (86.995, 3.81)
  line L612 (85.09, 3.175) -> (85.725, 3.81)
  line L613 (90.17, 1.905) -> (89.535, 1.27)
  line L614 (90.17, 3.175) -> (90.17, 1.905)
  line L615 (89.535, 3.81) -> (90.17, 3.175)
  line L616 (88.265, 3.81) -> (89.535, 3.81)
  arc A31 (22.225, 48.3344) -> (22.225, 48.6936) centre (22.225, 48.514) ccw
  arc A32 (22.225, 48.6936) -> (22.225, 48.3344) centre (22.225, 48.514) ccw
  line L617 (88.773, 47.244) -> (89.789, 48.26)
  line L618 (88.773, 33.528) -> (88.773, 47.244)
  line L619 (88.773, 11.303) -> (89.789, 10.287)
  line L620 (88.773, 22.987) -> (88.773, 11.303)
  line L621 (51.943, 8.128) -> (50.927, 7.112)
  line L622 (53.975, 8.128) -> (51.943, 8.128)
  line L623 (90.043, 8.128) -> (90.932, 7.239)
  line L624 (72.644, 8.128) -> (90.043, 8.128)
  line L625 (85.217, 41.021) -> (86.36, 42.164)
  line L626 (83.439, 41.021) -> (85.217, 41.021)
  line L627 (62.23, 41.021) -> (63.5, 41.021)
  line L628 (61.087, 42.164) -> (62.23, 41.021)
  line L629 (30.226, 45.085) -> (29.337, 45.974)
  line L630 (40.64, 45.085) -> (30.226, 45.085)
  line L631 (57.404, 45.085) -> (58.42, 46.101)
  line L632 (46.228, 45.085) -> (57.404, 45.085)
  line L633 (96.52, 52.705) -> (96.52, 52.07)
  line L634 (93.98, 52.705) -> (96.52, 52.705)
  line L635 (93.98, 52.07) -> (93.98, 52.705)
  line L636 (96.52, 5.207) -> (96.52, 5.715)
  line L637 (93.98, 5.207) -> (96.52, 5.207)
  line L638 (93.98, 5.715) -> (93.98, 5.207)
  line L639 (56.515, 49.53) -> (57.15, 50.165)
  line L640 (76.835, 52.07) -> (77.47, 51.435)
  line L641 (17.465, 6.194) -> (17.465, 5.894)
  line L642 (19.365, 6.194) -> (19.365, 5.894)
  line L643 (17.465, 12.394) -> (17.465, 12.094)
  line L644 (19.365, 12.394) -> (19.365, 12.094)
  line L645 (24.577, 12.394) -> (24.577, 12.094)
  line L646 (26.477, 12.394) -> (26.477, 12.094)
  line L647 (26.477, 6.194) -> (26.477, 5.894)
  line L648 (24.577, 6.194) -> (24.577, 5.894)
  line L649 (16.791, 22.635) -> (16.791, 20.035)
  line L650 (20.041, 22.635) -> (20.041, 20.035)
  line L651 (0, 52.3399) -> (0, 1) projected
  circle A33 centre (18.4152, 9.144) radius 3.0992
  circle A34 centre (25.5272, 9.144) radius 3.0992
  constraints: 1302 end point, 70 point on circle, 35 centre point, 21 point on line, 2 coincident, 2 concentric, 2 parallel, 2 tangent
extrude "Socket" add sketch "Sketch3" along normal blind 8.3 contours L4 L57 L56 L55 L5 A5 A6 A4 L60 L59 L58 | L54 L53 L52 L6 L63 L62 L61 A4 A5 L5 | L61 L5 A5 A4 | L51 L50 L49 L7 L66 L65 L64 L6 | L48 L47 L46 L8 L69 L68 L67 L7 | L45 L44 L43 L9 L72 L71 L70 L8 | L42 L41 L40 L10 L75 L74 L73 L9 | L39 L38 L37 L11 L78 L77 L76 L10 | L36 L35 L34 L12 L81 L80 L79 L11 | L33 L32 L31 L13 L84 L83 L82 L12 | L30 L29 L28 L14 L87 L86 L85 L13 | L27 L26 L25 L15 L90 L89 L88 L14 | L24 L23 L22 L16 L93 L92 L91 L15 | L113 L114 L115 L17 L96 L95 L94 L16 | L116 L117 L118 L18 L99 L98 L97 L17 | L119 L120 L121 L19 L102 L101 L100 L18 | L122 L123 L124 L20 L105 L104 L103 L19 | L125 L126 L127 L21 L108 L107 L106 L20 | L128 L129 L130 L112 L111 L110 L109 L21 | L161 L162 L214 L163 L167 L166 L165 L164 | L213 L203 L204 L209 L205 L216 L215 L214 | L208 L207 L206 L195 L212 L211 L210 L209 | L194 L193 L192 L200 L198 L197 L196 L195 | L199 L183 L184 L188 L639 L202 L201 L200 | L187 L186 L185 L175 L191 L190 L189 L188 | L174 L173 L172 L180 L178 L177 L176 L175 | L179 L168 L169 L171 L170 L182 L181 L180 | L217 L218 L271 L219 L223 L222 L221 L220 | L270 L260 L261 L266 L262 L273 L272 L271 | L265 L264 L263 L252 L269 L268 L267 L266 | L251 L250 L249 L257 L255 L254 L253 L252 | L256 L239 L240 L245 L241 L259 L258 L257 | L244 L243 L242 L231 L248 L247 L246 L245 | L230 L229 L228 L236 L234 L233 L232 L231 | L235 L224 L225 L227 L226 L238 L237 L236 | L290 L291 L357 L292 L296 L295 L294 L293 | L356 L355 L354 L346 L360 L359 L358 L357 | L345 L344 L343 L351 L349 L348 L347 L346 | L350 L333 L334 L339 L335 L353 L352 L351 | L338 L337 L336 L325 L342 L341 L340 L339 | L324 L323 L322 L330 L328 L327 L326 L325 | L329 L312 L313 L318 L314 L332 L331 L330 | L317 L316 L315 L304 L321 L320 L319 L318 | L303 L302 L301 L309 L307 L306 L305 L304 | L308 L297 L298 L300 L299 L311 L310 L309 | L447 L448 L500 L449 L453 L452 L451 L450 | L499 L489 L490 L495 L491 L502 L501 L500 | L494 L493 L492 L481 L498 L497 L496 L495 | L480 L479 L640 L486 L484 L483 L482 L481 | L485 L469 L470 L475 L471 L488 L487 L486 | L474 L473 L472 L461 L478 L477 L476 L475 | L460 L459 L458 L466 L464 L463 L462 L461 | L465 L454 L455 L457 L456 L468 L467 L466 | L503 L504 L557 L505 L509 L508 L507 L506 | L556 L546 L547 L552 L548 L559 L558 L557 | L551 L550 L549 L538 L555 L554 L553 L552 | L537 L536 L535 L543 L541 L540 L539 L538 | L542 L525 L526 L531 L527 L545 L544 L543 | L530 L529 L528 L517 L534 L533 L532 L531 | L516 L515 L514 L522 L520 L519 L518 L517 | L521 L510 L511 L513 L512 L524 L523 L522 | L560 L561 L614 L562 L566 L565 L564 L563 | L613 L603 L604 L609 L605 L616 L615 L614 | L608 L607 L606 L595 L612 L611 L610 L609 | L594 L593 L592 L600 L598 L597 L596 L595 | L599 L582 L583 L588 L584 L602 L601 L600 | L587 L586 L585 L574 L591 L590 L589 L588 | L573 L572 L571 L579 L577 L576 L575 L574 | L578 L567 L568 L570 L569 L581 L580 L579
extrude "Atmel2560" add sketch "Sketch3" along normal blind 1 contours L427 L434 L433 L432 L431 L430 L429 L428
extrude "Quarz1" add sketch "Sketch3" along normal blind 1 contours L0 A3 L1 A0 | L2 A2 L3 A1
extrude "Quarz2" add sketch "Sketch3" along normal blind 5 contours L0 A3 L1 A0
extrude "Extrusion7" add sketch "Sketch3" along normal blind 5 contours A34 A16 A15 | A33 A18 A17
extrude "Extrusion8" add sketch "Sketch3" along normal blind 1 contours A15 L646 L277 L276 L275 L274 L647 | L648 L281 L280 L279 L278 L645 A16 | A17 L644 L285 L284 L283 L282 L642 | L641 L289 L288 L287 L286 L643 A18 | A19 A20 L288 L289
extrude "Switch1" add sketch "Sketch3" along normal blind 2 contours L139 L158 L155 L156 L157 L159 L142 L149 L154 L153 L141 L160 L140 L146 L145 L144
extrude "Switch2" add sketch "Sketch3" along normal blind 4 contours A12 A11 | A14 A13
extrude "Pins1" add sketch "Sketch3" along normal blind 2.5 contours L363 L390 L386 L396 L383 L397 L393 L392 | L387 L385 L394 L384 L395 L386 L389 L363 | L380 L379 L378 L377 L381 L376 L382 L385 | L404 L407 L402 L401 L400 L399 L403 L398 | L416 L406 L417 L408 L411 L410 L409 L407 | L418 L405 L419 L415 L414 L413 L412 L408
sketch "Sketch4" plane through (0, 0, 2.5) normal (0, 0, 1) x (1, 0, 0)
  line L0 (15.113, 48.768) -> (16.383, 48.768) projected
  line L1 (17.653, 48.768) -> (18.923, 48.768) projected
  line L2 (20.193, 48.768) -> (21.463, 48.768) projected
  line L3 (16.383, 43.688) -> (15.113, 43.688) projected
  line L4 (18.923, 43.688) -> (17.653, 43.688) projected
  line L5 (21.463, 43.688) -> (20.193, 43.688) projected
  line L6 (67.437, 31.115) -> (67.437, 29.845) projected
  line L7 (62.357, 29.845) -> (62.357, 31.115) projected
  line L8 (62.357, 27.305) -> (62.357, 28.575) projected
  line L9 (67.437, 28.575) -> (67.437, 27.305) projected
  line L10 (67.437, 26.035) -> (67.437, 24.765) projected
  line L11 (62.357, 24.765) -> (62.357, 26.035) projected
  line L12 (62.357, 30.48) -> (67.437, 30.48) construction
  line L13 (62.357, 27.94) -> (67.437, 27.94) construction
  line L14 (62.357, 25.4) -> (67.437, 25.4) construction
  line L15 (20.828, 48.768) -> (20.828, 43.688) construction
  line L16 (18.288, 43.688) -> (18.288, 48.768) construction
  line L17 (15.748, 43.688) -> (15.748, 48.768) construction
  circle A0 centre (15.748, 47.478) radius 0.5
  circle A1 centre (15.748, 44.978) radius 0.5
  circle A2 centre (18.288, 47.478) radius 0.5
  circle A3 centre (18.288, 44.978) radius 0.5
  circle A4 centre (20.828, 47.478) radius 0.5
  circle A5 centre (20.828, 44.978) radius 0.5
  circle A6 centre (63.647, 30.48) radius 0.5
  circle A7 centre (66.147, 30.48) radius 0.5
  circle A8 centre (63.647, 27.94) radius 0.5
  circle A9 centre (66.147, 27.94) radius 0.5
  circle A10 centre (66.147, 25.4) radius 0.5
  circle A11 centre (63.647, 25.4) radius 0.5
  dimension "d95" = 1
  dimension "d96" = 1
  dimension "d97" = 2.5
  dimension "d98" = 1.29
  dimension "d99" = 1.29
  dimension "d100" = 2.5
  dimension "d101" = 1.29
  constraints: 12 centre point, 12 end point, 12 midpoint, 12 point on line, 10 equal radius, 4 horizontal alignment, 4 vertical alignment
  measures "d95" diameter of A0
  measures "d96" diameter of A1
  measures "d97" distance of A0.centre A1.centre
  measures "d98" distance from line of L3 A1.centre
  measures "d99" distance of L17.end A0.centre
  measures "d100" distance of A7.centre A6.centre
  measures "d101" distance of A7.centre L12.end
extrude "Pins2" add sketch "Sketch4" along normal blind 3.5
sketch "Sketch5" plane through (0, 0, 0) normal (0, 0, 1) x (1, 0, 0)
  line L0 (-1.8, 12.3) -> (11.7, 12.3)
  line L1 (11.7, 12.3) -> (11.7, 3.3)
  line L2 (11.7, 3.3) -> (-1.8, 3.3)
  line L3 (-1.8, 3.3) -> (-1.8, 12.3)
  line L4 (1, 0) -> (98.0599, 0) projected
  line L5 (0, 52.3399) -> (0, 1) projected
  dimension "d104" = 13.5
  dimension "d105" = 9
  dimension "d106" = 3.3
  dimension "d107" = 1.8
  constraints: 8 end point, 2 parallel, 1 horizontal, 1 perpendicular
  measures "d104" distance of L0.start L0.end
  measures "d105" distance of L2.end L0.start
  measures "d106" distance between parallel lines of L4 L2
  measures "d107" distance between parallel lines of L5 L3
extrude "Power" add sketch "Sketch5" along normal blind 11
sketch "Sketch6" plane through (-1.8, 3.3, 0) normal (-1, 0, 0) x (0, 0, 1)
  line L0 (11, 0) -> (11, 9) projected
  line L1 (0, 9) -> (11, 9) projected
  circle A0 centre (5.5, 4.5) radius 2.5
  point P0 (11, 4.5)
  point P1 (5.5, 9)
  dimension "d110" = 5
  constraints: 2 midpoint, 1 centre point, 1 horizontal alignment, 1 vertical alignment
  measures "d110" diameter of A0
extrude "Power2" cut sketch "Sketch6" against normal blind 10